LGR RM Front Holder (Goalie) (Autodesk Fusion 360 design; units mm, degrees)
Autodesk Fusion 360 part; units mm, degrees
sketch "Sketch1" plane through (0, 0, 0) normal (0, 0, 1) x (1, 0, 0)
  line L0 (28.55, 26.275) -> (30.55, 26.275)
  line L1 (30.55, 26.275) -> (30.55, -26.275)
  line L2 (30.55, -26.275) -> (28.55, -26.275)
  line L3 (28.55, -26.275) -> (28.55, 26.275)
  line L4 (-28.55, -26.275) -> (-30.55, -26.275)
  line L5 (-28.55, 26.275) -> (-28.55, -26.275)
  line L6 (-30.55, -26.275) -> (-30.55, 26.275)
  line L7 (-30.55, 26.275) -> (-28.55, 26.275)
  line L8 (-30.55, 26.275) -> (30.55, 26.275)
  line L9 (30.55, 26.275) -> (30.55, 28.275)
  line L10 (30.55, 28.275) -> (-30.55, 28.275)
  line L11 (-30.55, 28.275) -> (-30.55, 26.275)
  dimension "d1" = 2
  dimension "d2" = 52.55
  dimension "d4" = 26.275
  dimension "d5" = 2
  dimension "d6" = 52.55
  dimension "d7" = 57.1
  dimension "d8" = 28.55
  dimension "d9" = 2
  constraint horizontal L0
  constraint vertical L1
  constraint horizontal L2
  constraint vertical L3
  constraint horizontal L7
  constraint vertical L5
  constraint horizontal L4
  constraint vertical L6
  constraint horizontal L2.end L4.start
  constraint horizontal L8
  constraint vertical L9
  constraint horizontal L10
  constraint vertical L11
  constraint vertical L0.end L9.end
  measures "d1" distance of L1 L3
  measures "d2" distance of L0 L2
  measures "d4" distance of origin L0
  measures "d5" distance of L5 L6
  measures "d6" distance of L4 L7
  measures "d7" distance of L3 L5
  measures "d8" distance of origin L5
  measures "d9" distance of L8 L10
extrude "Extrude1" add sketch "Sketch1" along normal blind 20
sketch "Sketch2" plane through (0, 0, 20) normal (0, 0, 1) x (-1, 0, 0)
  line L0 (-30.55, 26.275) -> (-30.55, -28.275)
  line L1 (-30.55, -28.275) -> (30.55, -28.275)
  line L2 (30.55, -28.275) -> (30.55, 26.275)
  line L3 (30.55, 26.275) -> (28.55, 26.275)
  line L4 (28.55, 26.275) -> (28.55, -26.275)
  line L5 (28.55, -26.275) -> (-28.55, -26.275)
  line L6 (-28.55, -26.275) -> (-28.55, 26.275)
  line L7 (-28.55, 26.275) -> (-30.55, 26.275)
  line L8 (-30.55, 26.275) -> (-40.55, 26.275)
  line L9 (-40.55, 26.275) -> (-40.55, 16.275)
  line L10 (-40.55, 16.275) -> (-30.55, 16.275)
  line L11 (-30.55, 16.275) -> (-30.55, 26.275)
  line L12 (30.55, 26.275) -> (40.55, 26.275)
  line L13 (40.55, 26.275) -> (40.55, 16.275)
  line L14 (40.55, 16.275) -> (30.55, 16.275)
  line L15 (30.55, 16.275) -> (30.55, 26.275)
  dimension "d12" = 10
  dimension "d13" = 10
  dimension "d14" = 10
  dimension "d15" = 10
  constraint horizontal L8
  constraint vertical L9
  constraint horizontal L10
  constraint vertical L11
  constraint coincident L0.start L7.end
  constraint horizontal L12
  constraint vertical L13
  constraint horizontal L14
  constraint vertical L15
  constraint coincident L2.end L3.start
  measures "d12" distance of L8 L10
  measures "d13" distance of L9 L11
  measures "d14" distance of L12 L14
  measures "d15" distance of L13 L15
extrude "Extrude2" add sketch "Sketch2" against normal blind 20 contours L0 L8 L9 L10 L11 | L2 L12 L13 L14 L15
fillet "Fillet1" radius 2 2 edges at (40.55, -21.275, 0) (-40.55, -21.275, 0)
sketch "Sketch3" plane through (0, -16.275, 0) normal (0, 1, 0) x (-1, 0, 0)
  arc A0 (38.55, 0) -> (40.55, 2) centre (38.55, 2) ccw
  line L0 (40.55, 2) -> (40.55, 20)
  line L1 (40.55, 20) -> (30.55, 20)
  line L2 (30.55, 20) -> (30.55, 0)
  line L3 (30.55, 0) -> (38.55, 0)
  point P0 (34.75, 10)
  point P1 (-34.75, 10)
  dimension "d20" = 5.8
  dimension "d21" = 10
  dimension "d22" = 69.5
  constraint horizontal P0 P1
  measures "d20" distance of L0 P0
  measures "d21" distance of L3 P0
  measures "d22" distance of P0 P1
hole "Hole1" at (-34.75, -16.275, 10) at (34.75, -16.275, 10) direction (0, -1, 0) diameter 5.3 end through all counterbore diameter 10 counterbore depth 5
sketch "Sketch4" plane through (0, -16.275, 0) normal (0, 1, 0) x (-1, 0, 0)
  arc A0 (30.55, 7.2871) -> (30.55, 12.7129) centre (34.75, 10) ccw
  line L0 (30.55, 7.2871) -> (30.55, 0)
  line L1 (30.55, 0) -> (38.55, 0)
  arc A1 (38.55, 0) -> (40.55, 2) centre (38.55, 2) ccw
  line L2 (40.55, 2) -> (40.55, 20)
  line L3 (40.55, 20) -> (30.55, 20)
  line L4 (30.55, 20) -> (30.55, 12.7129)
  circle A2 centre (34.75, 10) radius 5
  circle A3 centre (-34.75, 10) radius 5
  dimension "d28" = 10
  dimension "d29" = 69.5
  constraint concentric A0 A2
  constraint coincident A0.end A2
  constraint horizontal A0.centre A3.centre
  measures "d28" diameter of A3
  measures "d29" distance of A0.centre A3.centre
extrude "Extrude3" cut sketch "Sketch4" along normal blind 7 contours A0 A2 | A3
sketch "Sketch5" plane through (0, 28.275, 0) normal (0, 1, 0) x (-1, 0, 0)
  line L0 (-30.55, 0) -> (30.55, 0)
  line L1 (30.55, 0) -> (30.55, 20)
  line L2 (30.55, 20) -> (-30.55, 20)
  line L3 (-30.55, 20) -> (-30.55, 0)
  line L4 (-20, 20) -> (20, 20)
  line L5 (20, 20) -> (20, 0)
  line L6 (20, 0) -> (-20, 0)
  line L7 (-20, 0) -> (-20, 20)
  dimension "d32" = 40
  dimension "d96" = 20
  constraint horizontal L4
  constraint vertical L5
  constraint horizontal L6
  constraint vertical L7
  constraint coincident L0 L5.end
  constraint coincident L2 L4.start
  measures "d32" distance of L5 L7
  measures "d96" distance of origin L7
extrude "Extrude4" add sketch "Sketch5" along normal blind 10 contours L0 L2 L4 L5 L6 L7
sketch "Sketch6" plane through (0, 0, 0) normal (0, 0, -1) x (1, 0, 0)
  line L0 (20, -38.275) -> (20, -28.275)
  line L1 (-30.55, -28.275) -> (-20, -28.275)
  line L2 (30.55, -28.275) -> (30.55, 16.275)
  line L3 (30.55, 16.275) -> (38.55, 16.275)
  line L4 (38.55, 16.275) -> (38.55, 26.275)
  line L5 (38.55, 26.275) -> (28.55, 26.275)
  line L6 (28.55, 26.275) -> (28.55, -26.275)
  line L7 (28.55, -26.275) -> (-28.55, -26.275)
  line L8 (-28.55, -26.275) -> (-28.55, 26.275)
  line L9 (-28.55, 26.275) -> (-38.55, 26.275)
  line L10 (-38.55, 26.275) -> (-38.55, 16.275)
  line L11 (-38.55, 16.275) -> (-30.55, 16.275)
  line L12 (-30.55, 16.275) -> (-30.55, -28.275)
  line L13 (-20, -28.275) -> (-20, -38.275)
  line L14 (-20, -38.275) -> (20, -38.275)
  line L15 (-28.55, -26.275) -> (-19.3, -26.275)
  line L16 (-19.3, -23.775) -> (-19.3, -22.025)
  line L17 (-24.3, -17.025) -> (-26.05, -17.025)
  line L18 (-28.55, -17.025) -> (-28.55, -26.275)
  line L19 (28.55, -26.275) -> (19.3, -26.275)
  line L20 (19.3, -23.775) -> (19.3, -22.025)
  line L21 (24.3, -17.025) -> (26.05, -17.025)
  line L22 (28.55, -17.025) -> (28.55, -26.275)
  arc A0 (-19.3, -22.025) -> (-24.3, -17.025) centre (-24.3, -22.025) ccw
  arc A1 (24.3, -17.025) -> (19.3, -22.025) centre (24.3, -22.025) ccw
  line L23 (28.55, -14.525) -> (28.55, -10)
  line L24 (-28.55, -14.525) -> (-28.55, -10)
  arc A2 (26.05, -17.025) -> (28.55, -14.525) centre (26.05, -14.525) ccw
  arc A3 (-28.55, -14.525) -> (-26.05, -17.025) centre (-26.05, -14.525) ccw
  line L25 (16.8, -26.275) -> (13, -26.275)
  line L26 (-16.8, -26.275) -> (-13, -26.275)
  arc A4 (16.8, -26.275) -> (19.3, -23.775) centre (16.8, -23.775) ccw
  arc A5 (-19.3, -23.775) -> (-16.8, -26.275) centre (-16.8, -23.775) ccw
  line L27 (20, -28.275) -> (30.55, -28.275)
  dimension "d38" = 9.25
  dimension "d39" = 9.25
  dimension "d40" = 9.25
  dimension "d41" = 9.25
  dimension "d42" = 5
  dimension "d43" = 5
  dimension "d44" = 2.5
  dimension "d45" = 2.5
  dimension "d46" = 2.5
  dimension "d47" = 2.5
  constraint horizontal L15
  constraint vertical L16
  constraint horizontal L17
  constraint vertical L18
  constraint coincident L7.end L8.start
  constraint horizontal L19
  constraint vertical L20
  constraint horizontal L21
  constraint vertical L22
  constraint coincident L6.end L7.start
  constraint tangent L17 A0
  constraint tangent L16 A0
  constraint tangent L21 A1
  constraint tangent L20 A1
  constraint coincident L6 L23.end
  constraint coincident L8 L24.end
  constraint coincident L22.start L21
  constraint coincident L22.start L23
  constraint tangent L21 A2
  constraint tangent L23 A2
  constraint coincident L18.start L24
  constraint coincident L18.start L17
  constraint tangent L24 A3
  constraint tangent L17 A3
  constraint coincident L7 L25.end
  constraint coincident L7 L26.end
  constraint coincident L19.end L25
  constraint coincident L19.end L20
  constraint tangent L25 A4
  constraint tangent L20 A4
  constraint coincident L15.end L26
  constraint coincident L15.end L16
  constraint tangent L26 A5
  constraint tangent L16 A5
  measures "d38" distance of L16 L18
  measures "d39" distance of L15 L17
  measures "d40" distance of L20 L22
  measures "d41" distance of L19 L21
  measures "d42" radius of A0
  measures "d43" radius of A1
  measures "d44" radius of A2
  measures "d45" radius of A3
  measures "d46" radius of A4
  measures "d47" radius of A5
extrude "Extrude5" add sketch "Sketch6" against normal blind 20 contours L6 L7 L19 L20 L21 L22 A1 A2 A4 | L7 L8 L15 L16 L17 L18 A0 A3 A5
sketch "Sketch7" plane through (0, 0, 20) normal (0, 0, 1) x (-1, 0, 0)
  line L0 (-30.55, -28.275) -> (-20, -28.275)
  line L1 (-20, -28.275) -> (20, -28.275)
  line L2 (30.55, -28.275) -> (30.55, 16.275)
  line L3 (30.55, 16.275) -> (40.55, 16.275)
  line L4 (40.55, 16.275) -> (40.55, 26.275)
  line L5 (40.55, 26.275) -> (28.55, 26.275)
  line L6 (28.55, 26.275) -> (28.55, -14.525)
  arc A0 (26.05, -17.025) -> (28.55, -14.525) centre (26.05, -14.525) ccw
  line L7 (26.05, -17.025) -> (24.3, -17.025)
  arc A1 (24.3, -17.025) -> (19.3, -22.025) centre (24.3, -22.025) ccw
  line L8 (19.3, -22.025) -> (19.3, -23.775)
  arc A2 (16.8, -26.275) -> (19.3, -23.775) centre (16.8, -23.775) ccw
  line L9 (16.8, -26.275) -> (-16.8, -26.275)
  arc A3 (-19.3, -23.775) -> (-16.8, -26.275) centre (-16.8, -23.775) ccw
  line L10 (-19.3, -23.775) -> (-19.3, -22.025)
  arc A4 (-19.3, -22.025) -> (-24.3, -17.025) centre (-24.3, -22.025) ccw
  line L11 (-24.3, -17.025) -> (-26.05, -17.025)
  arc A5 (-28.55, -14.525) -> (-26.05, -17.025) centre (-26.05, -14.525) ccw
  line L12 (-28.55, -14.525) -> (-28.55, 26.275)
  line L13 (-28.55, 26.275) -> (-40.55, 26.275)
  line L14 (-40.55, 26.275) -> (-40.55, 16.275)
  line L15 (-40.55, 16.275) -> (-30.55, 16.275)
  line L16 (-30.55, 16.275) -> (-30.55, -28.275)
  line L17 (20, -28.275) -> (30.55, -28.275)
  point P0 (24.05, -21.775)
  point P1 (-24.05, -21.775)
  dimension "d52" = 6.5
  dimension "d54" = 6.5
  constraint horizontal P0 P1
  measures "d52" distance of L2 P0
  measures "d54" distance of L16 P1
hole "Hole2" at (-24.05, 21.775, 20) at (24.05, 21.775, 20) direction (0, 0, -1) diameter 3 end through all
sketch "Sketch10" plane through (-30.55, 0, 0) normal (-1, 0, 0) x (0, -1, 0)
  line L0 (-28.275, 0) -> (16.275, 0)
  line L1 (16.275, 0) -> (16.275, 7.2871)
  line L2 (16.275, 7.2871) -> (9.275, 7.2871)
  line L3 (9.275, 7.2871) -> (9.275, 12.7129)
  line L4 (9.275, 12.7129) -> (16.275, 12.7129)
  line L5 (16.275, 12.7129) -> (16.275, 20)
  line L6 (16.275, 20) -> (-28.275, 20)
  line L7 (-11.225, 15.2411) -> (-11.225, 4.8453)
  line L8 (13.275, 15.2453) -> (13.275, 4.8411)
  line L9 (-28.275, 20) -> (-28.275, 0)
  line L10 (-6.5475, 18) -> (8.5844, 18)
  line L11 (-6.5475, 2) -> (8.5844, 2)
  line L12 (-7.0853, 3.8431) -> (0.4635, 8.6578)
  line L13 (1.5372, 8.6589) -> (9.1204, 3.8442)
  line L14 (11.7503, 3.9899) -> (3.3712, 9.1548)
  line L15 (3.3657, 10.854) -> (11.7448, 16.0932)
  line L16 (9.1204, 16.1558) -> (1.5372, 11.3411)
  line L17 (0.4635, 11.3422) -> (-7.0853, 16.1569)
  line L18 (-9.6931, 16.0879) -> (-1.358, 10.8529)
  line L19 (-1.3634, 9.1558) -> (-9.6986, 3.9951)
  arc A0 (-9.6931, 16.0879) -> (-11.225, 15.2411) centre (-10.225, 15.2411) ccw
  arc A1 (-11.225, 4.8453) -> (-9.6986, 3.9951) centre (-10.225, 4.8453) ccw
  arc A2 (-1.3634, 9.1558) -> (-1.358, 10.8529) centre (-1.8898, 10.0061) ccw
  arc A3 (1.5372, 8.6589) -> (0.4635, 8.6578) centre (1.0012, 7.8147) ccw
  arc A4 (8.5844, 2) -> (9.1204, 3.8442) centre (8.5844, 3) ccw
  arc A5 (-7.0853, 3.8431) -> (-6.5475, 2) centre (-6.5475, 3) ccw
  arc A6 (11.7503, 3.9899) -> (13.275, 4.8411) centre (12.275, 4.8411) ccw
  arc A7 (13.275, 15.2453) -> (11.7448, 16.0932) centre (12.275, 15.2453) ccw
  arc A8 (9.1204, 16.1558) -> (8.5844, 18) centre (8.5844, 17) ccw
  arc A9 (-6.5475, 18) -> (-7.0853, 16.1569) centre (-6.5475, 17) ccw
  arc A10 (0.4635, 11.3422) -> (1.5372, 11.3411) centre (1.0012, 12.1853) ccw
  arc A11 (3.3657, 10.854) -> (3.3712, 9.1548) centre (3.8959, 10.0061) ccw
  line L20 (-28.275, 20) -> (-28.275, 0)
  point P0 (-11.225, 17.05)
  point P1 (-11.225, 3.05)
  point P2 (13.275, 17.05)
  point P3 (13.275, 3.05)
  point P4 (-9.975, 18)
  point P5 (12.025, 18)
  point P6 (-9.975, 2)
  point P7 (12.025, 2)
  point P8 (1.025, 10.05)
  point P9 (1, 9)
  point P10 (0, 10)
  point P11 (1, 11)
  point P12 (2, 10)
  dimension "d77" = 3
  dimension "d78" = 17.05
  dimension "d79" = 2
  dimension "d80" = 2
  dimension "d81" = 11
  dimension "d82" = 7
  dimension "d83" = 22
  dimension "d84" = 22
  dimension "d85" = 14
  dimension "d86" = 14
  dimension "d87" = 4.25
  dimension "d88" = 3.05
  dimension "d89" = 1
  constraint perpendicular L6 L7
  constraint vertical L8
  constraint horizontal L10
  constraint perpendicular L7 L11
  constraint horizontal P0 P2
  constraint vertical P4 P6
  constraint coincident P0 L18
  constraint coincident P0 L7
  constraint tangent L18 A0
  constraint tangent L7 A0
  constraint coincident P1 L7
  constraint coincident P1 L19
  constraint tangent L7 A1
  constraint tangent L19 A1
  constraint equal A0 A1
  constraint tangent L19 A2
  constraint tangent L18 A2
  constraint equal A0 A2
  constraint tangent L12 A3
  constraint tangent L13 A3
  constraint equal A0 A3
  constraint coincident P7 L13
  constraint coincident P7 L11
  constraint tangent L13 A4
  constraint tangent L11 A4
  constraint equal A0 A4
  constraint coincident P6 L11
  constraint coincident P6 L12
  constraint tangent L11 A5
  constraint tangent L12 A5
  constraint equal A0 A5
  constraint coincident P3 L14
  constraint coincident P3 L8
  constraint tangent L14 A6
  constraint tangent L8 A6
  constraint equal A0 A6
  constraint coincident P2 L8
  constraint coincident P2 L15
  constraint tangent L8 A7
  constraint tangent L15 A7
  constraint equal A0 A7
  constraint coincident P5 L16
  constraint coincident P5 L10
  constraint tangent L16 A8
  constraint tangent L10 A8
  constraint equal A0 A8
  constraint coincident P4 L17
  constraint coincident P4 L10
  constraint tangent L17 A9
  constraint tangent L10 A9
  constraint equal A0 A9
  constraint tangent L16 A10
  constraint tangent L17 A10
  constraint equal A0 A10
  constraint tangent L14 A11
  constraint tangent L15 A11
  constraint equal A0 A11
  measures "d77" distance of L5 L8
  measures "d78" distance of L7 L9
  measures "d79" distance of L6 L10
  measures "d80" distance of L0 L11
  measures "d81" horizontal distance of P5 P8
  measures "d82" vertical distance of P2 P8
  measures "d83" distance of P4 P5
  measures "d84" distance of P6 P7
  measures "d85" distance of P2 P3
  measures "d86" distance of P0 P1
  measures "d87" distance of L5 P5
  measures "d88" distance of L0 P3
  measures "d89" radius of A0
extrude "Extrude8" cut sketch "Sketch10" against normal blind 65 contours L2 L3 L4 L8 L14 L15 A6 A7 A11 | L2 L3 L4 L8 | L7 L18 L19 A0 A1 A2 | L10 L16 L17 A8 A9 A10 | L11 L12 L13 A3 A4 A5
extrude "Extrude9" cut 2 faces at (27.0333, 28.275, 6.6667) (-23.5167, 28.275, 13.3333) along direction (0, -1, 0) blind 1.55
extrude "Extrude10" cut 1 faces at (-6.6667, 38.275, 13.3333) along direction (0, -1, 0) blind 4.5
fillet "Fillet4" radius 2.5 6 edges at (-20, 26.725, 10) (-20, 33.775, 10) (-30.55, 26.725, 10) (20, 33.775, 10) (20, 26.725, 10) (30.55, 26.725, 10)
sketch "Sketch11" plane through (0, 33.775, 0) normal (0, 1, 0) x (-1, 0, 0)
  line L0 (-17.5, 20) -> (-17.5, 0)
  line L1 (-17.5, 0) -> (17.5, 0)
  line L2 (17.5, 0) -> (17.5, 20)
  line L3 (17.5, 20) -> (-17.5, 20)
  line L4 (-22.5, 4.5) -> (22.5, 4.5)
  line L5 (22.5, 4.5) -> (22.5, 20)
  line L6 (22.5, 20) -> (-22.5, 20)
  line L7 (-22.5, 20) -> (-22.5, 4.5)
  dimension "d99" = 4.5
  dimension "d100" = 45
  dimension "d101" = 15.5
  dimension "d102" = 22.5
  constraint horizontal L4
  constraint vertical L5
  constraint horizontal L6
  constraint vertical L7
  measures "d99" distance of L1 L4
  measures "d100" distance of L5 L7
  measures "d101" distance of L4 L6
  measures "d102" distance of origin L7
extrude "Extrude11" cut sketch "Sketch11" against normal blind 7.05 contours L0 L2 L3 L4 L6 | L0 L4 L6 L7 | L2 L4 L5 L6
fillet "Fillet7" radius 2 1 edges at (0, 26.725, 4.5)
sketch "Sketch15" plane through (0, 26.725, 0) normal (0, 1, 0) x (-1, 0, 0)
  line L0 (-22.5, 0) -> (-22.5, 6.5)
  line L1 (-22.5, 6.5) -> (22.5, 6.5)
  line L2 (22.5, 6.5) -> (22.5, 0)
  line L3 (22.5, 0) -> (28.05, 0)
  line L4 (28.05, 0) -> (28.05, 20)
  line L5 (28.05, 20) -> (-28.05, 20)
  line L6 (-28.05, 20) -> (-28.05, 0)
  line L7 (-28.05, 0) -> (-22.5, 0)
  line L8 (22.5, 6.5) -> (-22.5, 6.5)
  line L9 (-22.5, 6.5) -> (-22.5, 0)
  line L10 (-22.5, 0) -> (22.5, 0)
  line L11 (22.5, 0) -> (22.5, 6.5)
  constraint horizontal L8
  constraint vertical L9
  constraint horizontal L10
  constraint vertical L11
  constraint coincident L0.start L7.end
  constraint coincident L1.end L2.start
extrude "Extrude15" cut sketch "Sketch15" along normal blind 15 contours L0 L1 L2 L8 L9 L10 L11
sketch "Sketch16" plane through (0, 0, 0) normal (0, 0, -1) x (1, 0, 0)
  circle A0 centre (24.05, -21.775) radius 1.5
  circle A1 centre (-24.05, -21.775) radius 1.5
  line L0 (-28.05, -26.725) -> (28.05, -26.725)
  arc A2 (28.05, -26.725) -> (30.55, -24.225) centre (28.05, -24.225) ccw
  line L1 (30.55, -24.225) -> (30.55, 16.275)
  line L2 (30.55, 16.275) -> (38.55, 16.275)
  line L3 (38.55, 16.275) -> (38.55, 26.275)
  line L4 (38.55, 26.275) -> (28.55, 26.275)
  line L5 (28.55, 26.275) -> (28.55, -14.525)
  arc A3 (26.05, -17.025) -> (28.55, -14.525) centre (26.05, -14.525) ccw
  line L6 (26.05, -17.025) -> (24.3, -17.025)
  arc A4 (24.3, -17.025) -> (19.3, -22.025) centre (24.3, -22.025) ccw
  line L7 (19.3, -22.025) -> (19.3, -23.775)
  arc A5 (16.8, -26.275) -> (19.3, -23.775) centre (16.8, -23.775) ccw
  line L8 (16.8, -26.275) -> (-16.8, -26.275)
  arc A6 (-19.3, -23.775) -> (-16.8, -26.275) centre (-16.8, -23.775) ccw
  line L9 (-19.3, -23.775) -> (-19.3, -22.025)
  arc A7 (-19.3, -22.025) -> (-24.3, -17.025) centre (-24.3, -22.025) ccw
  line L10 (-24.3, -17.025) -> (-26.05, -17.025)
  arc A8 (-28.55, -14.525) -> (-26.05, -17.025) centre (-26.05, -14.525) ccw
  line L11 (-28.55, -14.525) -> (-28.55, 26.275)
  line L12 (-28.55, 26.275) -> (-38.55, 26.275)
  line L13 (-38.55, 26.275) -> (-38.55, 16.275)
  line L14 (-38.55, 16.275) -> (-30.55, 16.275)
  line L15 (-30.55, 16.275) -> (-30.55, -24.225)
  arc A9 (-30.55, -24.225) -> (-28.05, -26.725) centre (-28.05, -24.225) ccw
  line L16 (25.55, -17.025) -> (24.3, -17.025)
  line L17 (-30.55, -22.025) -> (-30.55, -24.225)
  line L18 (-28.05, -26.725) -> (28.05, -26.725)
  line L19 (30.55, -24.225) -> (30.55, -22.025)
  line L20 (19.3, -23.775) -> (19.3, -22.025)
  line L21 (-19.3, -23.775) -> (-19.3, -22.025)
  arc A10 (28.05, -26.725) -> (30.55, -24.225) centre (28.05, -24.225) ccw
  arc A11 (-30.55, -24.225) -> (-28.05, -26.725) centre (-28.05, -24.225) ccw
  arc A12 (24.3, -17.025) -> (19.3, -22.025) centre (24.3, -22.025) ccw
  line L22 (-24.3, -17.025) -> (-25.55, -17.025)
  arc A13 (-19.3, -22.025) -> (-24.3, -17.025) centre (-24.3, -22.025) ccw
  line L23 (16.8, -26.275) -> (-16.8, -26.275)
  arc A14 (16.8, -26.275) -> (19.3, -23.775) centre (16.8, -23.775) ccw
  arc A15 (-19.3, -23.775) -> (-16.8, -26.275) centre (-16.8, -23.775) ccw
  circle A16 centre (24.05, -21.775) radius 1.5
  circle A17 centre (-24.05, -21.775) radius 1.5
  arc A18 (-25.55, -17.025) -> (-30.55, -22.025) centre (-25.55, -22.025) ccw
  arc A19 (30.55, -22.025) -> (25.55, -17.025) centre (25.55, -22.025) ccw
  dimension "d168" = 61.1
  dimension "d169" = 9.7
  dimension "d170" = 38.6
  dimension "d171" = 11.25
  dimension "d172" = 2.5
  dimension "d173" = 5
  dimension "d174" = 5
  dimension "d175" = 0.45
  dimension "d176" = 2.5
  dimension "d177" = 2.5
  dimension "d178" = 5
  dimension "d179" = 5
  constraint horizontal L16
  constraint vertical L17
  constraint horizontal L18
  constraint vertical L19
  constraint perpendicular L16 L20
  constraint perpendicular L16 L21
  constraint tangent L19 A10
  constraint tangent L18 A10
  constraint tangent L18 A11
  constraint tangent L17 A11
  constraint equal A10 A11
  constraint tangent L16 A12
  constraint tangent L20 A12
  constraint tangent L21 A13
  constraint tangent L22 A13
  constraint perpendicular L21 L23
  constraint tangent L23 A14
  constraint tangent L20 A14
  constraint tangent L21 A15
  constraint tangent L23 A15
  constraint concentric A0 A16
  constraint concentric A1 A17
  constraint tangent L22 A18
  constraint tangent L17 A18
  constraint tangent L19 A19
  constraint tangent L16 A19
  measures "d168" distance of L17 L19
  measures "d169" distance of L16 L18
  measures "d170" distance of L20 L21
  measures "d171" distance of L19 L20
  measures "d172" radius of A10
  measures "d173" radius of A12
  measures "d174" radius of A13
  measures "d175" distance of L18 L23
  measures "d176" radius of A14
  measures "d177" radius of A15
  measures "d178" radius of A18
  measures "d179" radius of A19
extrude "Extrude16" add sketch "Sketch16" along normal blind 20 contours L0 A2 L1 L6 A4 L7 A5 L8 A6 L9 A7 L10 L15 A9 L16 L17 L18 L19 L20 L21 A10 A11 A12 L22 A13 L23 A14 A15 A18 A19
sketch "Sketch18" plane through (0, 0, 20) normal (0, 0, 1) x (-1, 0, 0)
  line L0 (-28.05, -26.725) -> (28.05, -26.725)
  arc A0 (28.05, -26.725) -> (30.55, -24.225) centre (28.05, -24.225) ccw
  line L1 (30.55, -24.225) -> (30.55, 16.275)
  line L2 (30.55, 16.275) -> (40.55, 16.275)
  line L3 (40.55, 16.275) -> (40.55, 26.275)
  line L4 (40.55, 26.275) -> (28.55, 26.275)
  line L5 (28.55, 26.275) -> (28.55, -14.525)
  arc A1 (26.05, -17.025) -> (28.55, -14.525) centre (26.05, -14.525) ccw
  line L6 (26.05, -17.025) -> (24.3, -17.025)
  arc A2 (24.3, -17.025) -> (19.3, -22.025) centre (24.3, -22.025) ccw
  line L7 (19.3, -22.025) -> (19.3, -23.775)
  arc A3 (16.8, -26.275) -> (19.3, -23.775) centre (16.8, -23.775) ccw
  line L8 (16.8, -26.275) -> (-16.8, -26.275)
  arc A4 (-19.3, -23.775) -> (-16.8, -26.275) centre (-16.8, -23.775) ccw
  line L9 (-19.3, -23.775) -> (-19.3, -22.025)
  arc A5 (-19.3, -22.025) -> (-24.3, -17.025) centre (-24.3, -22.025) ccw
  line L10 (-24.3, -17.025) -> (-26.05, -17.025)
  arc A6 (-28.55, -14.525) -> (-26.05, -17.025) centre (-26.05, -14.525) ccw
  line L11 (-28.55, -14.525) -> (-28.55, 26.275)
  line L12 (-28.55, 26.275) -> (-40.55, 26.275)
  line L13 (-40.55, 26.275) -> (-40.55, 16.275)
  line L14 (-40.55, 16.275) -> (-30.55, 16.275)
  line L15 (-30.55, 16.275) -> (-30.55, -24.225)
  arc A7 (-30.55, -24.225) -> (-28.05, -26.725) centre (-28.05, -24.225) ccw
  circle A8 centre (24.05, -21.775) radius 1.5
  circle A9 centre (-24.05, -21.775) radius 1.5
  line L16 (19.3, -23.775) -> (-19.3, -23.775)
  line L17 (-19.3, -23.775) -> (-19.3, -26.725)
  line L18 (-19.3, -26.725) -> (19.3, -26.725)
  line L19 (19.3, -26.725) -> (19.3, -23.775)
  dimension "d192" = 2.95
  dimension "d193" = 38.6
  constraint horizontal L16
  constraint vertical L17
  constraint horizontal L18
  constraint vertical L19
  constraint coincident L7.end A3.end
  measures "d192" distance of L16 L18
  measures "d193" distance of L17 L19
extrude "Extrude17" cut sketch "Sketch18" against normal blind 10 contours L0 A3 L8 A4 L17 L18 L19
fillet "Fillet8" radius 2.5 2 edges at (-19.3, 26.725, 15) (19.3, 26.725, 15)
fillet "Fillet9" radius 2.5 4 edges at (20.0322, 25.9928, 10) (19.3, 24, 10) (-19.3, 24, 10) (-20.0322, 25.9928, 10)
fillet "Fillet10" radius 15 2 edges at (29.0855, 18.4895, 0) (-29.0855, 18.4895, 0)
sketch "Sketch20" plane through (0, 26.725, 0) normal (0, 1, 0) x (-1, 0, 0)
  line L0 (-21.8, 12.5) -> (-21.8, 20)
  line L1 (-21.8, 20) -> (-28.05, 20)
  line L2 (-28.05, 20) -> (-28.05, -20)
  line L3 (-28.05, -20) -> (28.05, -20)
  line L4 (28.05, -20) -> (28.05, 20)
  line L5 (28.05, 20) -> (21.8, 20)
  line L6 (21.8, 20) -> (21.8, 12.5)
  spline S0 degree 3 poles (17.4699, 10) (17.7885, 10) (18.1326, 10.0486) (18.7976, 10.2365) (19.1187, 10.3749) (19.8306, 10.7581) (20.2629, 11.0723) (21.0731, 11.7716) (21.4536, 12.1536) (21.8, 12.5) knots 1.263831 1.263831 1.263831 1.263831 1.35941 1.35941 1.454989 1.454989 1.601942 1.601942 1.748896 1.748896 1.748896 1.748896
  line L7 (17.4699, 10) -> (-17.4699, 10)
  spline S1 degree 3 poles (-21.8, 12.5) (-21.4536, 12.1536) (-21.0731, 11.7716) (-20.2629, 11.0723) (-19.8306, 10.7581) (-19.1187, 10.3749) (-18.7976, 10.2365) (-18.1326, 10.0486) (-17.7885, 10) (-17.4699, 10) knots 0 0 0 0 0.146954 0.146954 0.293907 0.293907 0.389486 0.389486 0.485065 0.485065 0.485065 0.485065
  line L8 (20, -20) -> (-20, -20)
  line L9 (-20, -20) -> (-20, -15)
  line L10 (-20, -15) -> (20, -15)
  line L11 (20, -15) -> (20, -20)
  dimension "d224" = 5
  dimension "d225" = 40
  dimension "d226" = 20
  constraint horizontal L8
  constraint vertical L9
  constraint horizontal L10
  constraint vertical L11
  constraint coincident L3 L8.start
  measures "d224" distance of L8 L10
  measures "d225" distance of L9 L11
  measures "d226" distance of origin L9
extrude "Extrude19" add sketch "Sketch20" along normal blind 7.05 contours L3 L8 L9 L10 L11
fillet "Fillet11" radius 2.5 2 edges at (-20, 26.725, -17.5) (-20, 33.775, -17.5)
fillet "Fillet11" radius 2.5 2 edges at (20, 33.775, -17.5) (20, 26.725, -17.5)
fillet "Fillet12" radius 2.5 1 edges at (0, 26.725, -15)
sketch "Sketch21" plane through (0, 26.725, 0) normal (0, 1, 0) x (-1, 0, 0)
  line L0 (22.5, -12.5) -> (22.5, -20)
  line L1 (22.5, -20) -> (28.05, -20)
  line L2 (28.05, -20) -> (28.05, 20)
  line L3 (28.05, 20) -> (21.8, 20)
  line L4 (21.8, 20) -> (21.8, 12.5)
  spline S0 degree 3 poles (17.4699, 10) (17.7885, 10) (18.1326, 10.0486) (18.7976, 10.2365) (19.1187, 10.3749) (19.8306, 10.7581) (20.2629, 11.0723) (21.0731, 11.7716) (21.4536, 12.1536) (21.8, 12.5) knots 1.263831 1.263831 1.263831 1.263831 1.35941 1.35941 1.454989 1.454989 1.601942 1.601942 1.748896 1.748896 1.748896 1.748896
  line L5 (17.4699, 10) -> (-17.4699, 10)
  spline S1 degree 3 poles (-21.8, 12.5) (-21.4536, 12.1536) (-21.0731, 11.7716) (-20.2629, 11.0723) (-19.8306, 10.7581) (-19.1187, 10.3749) (-18.7976, 10.2365) (-18.1326, 10.0486) (-17.7885, 10) (-17.4699, 10) knots 0 0 0 0 0.146954 0.146954 0.293907 0.293907 0.389486 0.389486 0.485065 0.485065 0.485065 0.485065
  line L6 (-21.8, 12.5) -> (-21.8, 20)
  line L7 (-21.8, 20) -> (-28.05, 20)
  line L8 (-28.05, 20) -> (-28.05, -20)
  line L9 (-28.05, -20) -> (-22.5, -20)
  line L10 (-22.5, -20) -> (-22.5, -12.5)
  line L11 (-22.5, -12.5) -> (22.5, -12.5)
  line L12 (16.8, -6.4222) -> (16.8, 3.9222)
  line L13 (-16.8, -6.4222) -> (-16.8, 3.9222)
  line L14 (12.6427, 7.5) -> (-12.6427, 7.5)
  line L15 (12.6427, -10) -> (-12.6427, -10)
  line L16 (-19.3, 12.5) -> (-19.3, 20)
  line L17 (19.3, 20) -> (19.3, 12.5)
  line L18 (12.8627, 6.551) -> (1.3198, 0.8965)
  line L19 (-1.3198, 0.8965) -> (-12.8627, 6.551)
  line L20 (-15.3731, 4.8265) -> (-4.4158, -0.3457)
  line L21 (-4.4158, -2.1543) -> (-15.3731, -7.3265)
  line L22 (-12.8627, -9.051) -> (-1.3198, -3.3965)
  line L23 (1.3198, -3.3965) -> (12.8627, -9.051)
  line L24 (15.3731, -7.3265) -> (4.4158, -2.1543)
  line L25 (4.4158, -0.3457) -> (15.3731, 4.8265)
  arc A0 (4.4158, -0.3457) -> (4.4158, -2.1543) centre (4.8427, -1.25) ccw
  arc A1 (-4.4158, -2.1543) -> (-4.4158, -0.3457) centre (-4.8427, -1.25) ccw
  arc A2 (-1.3198, 0.8965) -> (1.3198, 0.8965) centre (0, 3.5906) ccw
  arc A3 (1.3198, -3.3965) -> (-1.3198, -3.3965) centre (0, -6.0906) ccw
  arc A4 (12.6427, -10) -> (12.8627, -9.051) centre (12.6427, -9.5) ccw
  arc A5 (-12.8627, -9.051) -> (-12.6427, -10) centre (-12.6427, -9.5) ccw
  arc A6 (-12.6427, 7.5) -> (-12.8627, 6.551) centre (-12.6427, 7) ccw
  arc A7 (12.8627, 6.551) -> (12.6427, 7.5) centre (12.6427, 7) ccw
  arc A8 (15.3731, -7.3265) -> (16.8, -6.4222) centre (15.8, -6.4222) ccw
  arc A9 (16.8, 3.9222) -> (15.3731, 4.8265) centre (15.8, 3.9222) ccw
  arc A10 (-15.3731, 4.8265) -> (-16.8, 3.9222) centre (-15.8, 3.9222) ccw
  arc A11 (-16.8, -6.4222) -> (-15.3731, -7.3265) centre (-15.8, -6.4222) ccw
  point P0 (-16.8, -8)
  point P1 (-16.8, 5.5)
  point P2 (14.8, 7.5)
  point P3 (-14.8, 7.5)
  point P4 (-14.8, -10)
  point P5 (0, -2.75)
  point P6 (0, 0.25)
  point P7 (-2.5, -1.25)
  point P8 (2.5, -1.25)
  dimension "d235" = 2.5
  dimension "d236" = 2.5
  dimension "d237" = 2.5
  dimension "d238" = 2.5
  dimension "d239" = 3
  dimension "d240" = 5
  dimension "d241" = 2.5
  dimension "d243" = 7.25
  dimension "d244" = 1.5
  dimension "d245" = 2
  dimension "d246" = 2
  dimension "d247" = 2
  dimension "d248" = 2
  dimension "d249" = 1
  dimension "d250" = 3
  dimension "d251" = 0.5
  dimension "d252" = 1
  constraint perpendicular L11 L12
  constraint vertical L13
  constraint horizontal L14
  constraint horizontal L15
  constraint vertical P5 P6
  constraint vertical origin P5
  constraint horizontal P7 P8
  constraint vertical P3 P4
  constraint tangent L24 A0
  constraint tangent L25 A0
  constraint tangent L21 A1
  constraint tangent L20 A1
  constraint equal A0 A1
  constraint tangent L18 A2
  constraint tangent L19 A2
  constraint tangent L23 A3
  constraint tangent L22 A3
  constraint equal A2 A3
  constraint tangent L23 A4
  constraint tangent L15 A4
  constraint coincident P4 L15
  constraint coincident P4 L22
  constraint tangent L15 A5
  constraint tangent L22 A5
  constraint equal A4 A5
  constraint coincident P3 L19
  constraint coincident P3 L14
  constraint tangent L19 A6
  constraint tangent L14 A6
  constraint equal A4 A6
  constraint coincident P2 L14
  constraint coincident P2 L18
  constraint tangent L14 A7
  constraint tangent L18 A7
  constraint equal A4 A7
  constraint tangent L24 A8
  constraint tangent L12 A8
  constraint tangent L12 A9
  constraint tangent L25 A9
  constraint equal A8 A9
  constraint coincident P1 L20
  constraint coincident P1 L13
  constraint tangent L20 A10
  constraint tangent L13 A10
  constraint equal A8 A10
  constraint coincident P0 L13
  constraint coincident P0 L21
  constraint tangent L13 A11
  constraint tangent L21 A11
  constraint equal A8 A11
  measures "d235" distance of L11 L15
  measures "d236" distance of L5 L14
  measures "d237" distance of L13 L16
  measures "d238" distance of L12 L17
  measures "d239" distance of P5 P6
  measures "d240" distance of P7 P8
  measures "d241" horizontal distance of origin P7
  measures "d243" distance of L14 P6
  measures "d244" vertical distance of P6 P7
  measures "d245" distance of L12 P2
  measures "d246" horizontal distance of P1 P3
  measures "d247" vertical distance of P0 P4
  measures "d248" vertical distance of P1 P3
  measures "d249" radius of A0
  measures "d250" radius of A2
  measures "d251" radius of A4
  measures "d252" radius of A8
extrude "Extrude20" cut sketch "Sketch21" against normal blind 0.45 contours L12 L24 L25 A0 A8 A9 | L13 L20 L21 A1 A10 A11 | L14 L18 L19 A2 A6 A7 | L15 L22 L23 A3 A4 A5
equation "d4 = ( 52.55 / 2 ) * 1 mm"
equation "d8 = ( 57.1 / 2 ) * 1 mm"
equation "d20 = 3.75 mm + 2.5 mm - 0.45 mm"
equation "d88 = ( ( 20.1 - 14 ) / 2 ) * 1 mm"
equation "d102 = ( 45 / 2 ) * 1 mm"
equation "d243 = ( ( 17.5 - 3 ) / 2 ) * 1 mm"
